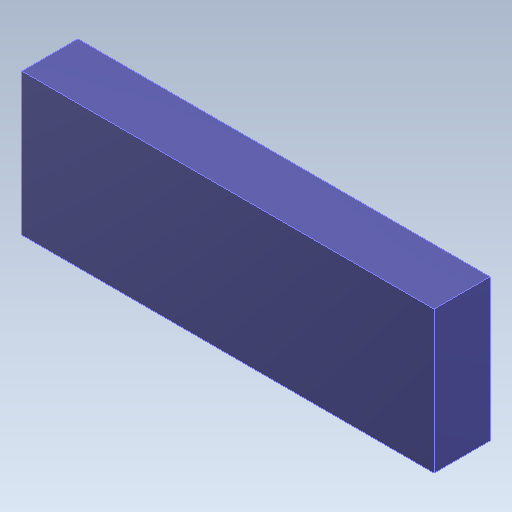
# Autodesk Inventor part: C050-025X075
Saved by Autodesk Inventor 2021 (Build 250183000, 183)
## iProperties
Created: 2020-11-18
Part Number: C050-025X075
Material: Generic
Document SubType Name: Modeling
Designer: Admin
Density: 1 g/cm^3
Appearance: C050-025X075, C050-025X075
Author: Admin
Autodesk Inventor part; units mm, degrees
ref_plane "YZ Plane" through (0, 0, 0) normal (1, 0, 0) x (0, 1, 0)
ref_plane "XZ Plane" through (0, 0, 0) normal (0, 1, 0) x (-1, 0, 0)
ref_plane "XY Plane" through (0, 0, 0) normal (0, 0, 1) x (1, 0, 0)
sketch "C050-025X075, C050-025X075_1" plane through (0, 0, 0) normal (0, 0, 1) x (1, 0, 0)
  line L0 (-3.683, 1.27) -> (3.683, 1.27)
  line L1 (3.683, 1.27) -> (3.683, -1.27)
  line L2 (3.683, -1.27) -> (-3.683, -1.27)
  line L3 (-3.683, -1.27) -> (-3.683, 1.27)
  constraints: 8 end point
extrude "Extrusion1" add sketch "C050-025X075, C050-025X075_1" along normal blind 1
body "Solid1"
